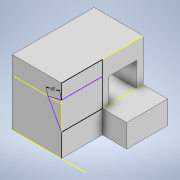
# Autodesk Inventor part: Vỏ
Saved by Autodesk Inventor 2020 (Build 240168000, 168)
## iProperties
Created: 2022-09-23
Part Number: Vỏ
Material: Generic
Document SubType Name: Modeling
Designer: ASUS
Density: 1 g/cm^3
Appearance: Default
Author: ASUS
Autodesk Inventor part; units mm, degrees
ref_plane "YZ Plane" through (0, 0, 0) normal (1, 0, 0) x (0, 1, 0)
ref_plane "XZ Plane" through (0, 0, 0) normal (0, 1, 0) x (-1, 0, 0)
ref_plane "XY Plane" through (0, 0, 0) normal (0, 0, 1) x (1, 0, 0)
sketch "Sketch1" plane through (0, 0, 0) normal (1, 0, 0) x (0, 1, 0)
  line L0 (0, 0) -> (400, 0)
  line L1 (400, 0) -> (400, -500)
  line L2 (400, -500) -> (0, -500)
  line L3 (0, -500) -> (0, 0)
  dimension "d0" = 400
  dimension "d1" = 500
  constraints: 8 end point, 2 parallel, 1 horizontal, 1 perpendicular
  measures "d0" distance of L1.end L2.end
  measures "d1" distance of L0.end L1.end
extrude "Extrusion1" add sketch "Sketch1" against normal blind 300
sketch "Sketch2" plane through (0, 0, 0) normal (1, 0, 0) x (0, 0, -1)
  line L0 (500, 0) -> (0, 0) projected
  line L1 (500, 400) -> (500, 0) projected
  line L2 (250, 0) -> (500, 0)
  line L3 (500, 0) -> (500, 140)
  line L4 (500, 140) -> (250, 140)
  line L5 (250, 140) -> (250, 0)
  dimension "d4" = 140
  constraints: 8 end point, 2 parallel, 1 horizontal, 1 midpoint, 1 perpendicular, 1 point on line
  measures "d4" distance of L3.end L2.end
extrude "Extrusion2" add sketch "Sketch2" along normal blind 150
sketch "Sketch3" plane through (0, 0, 0) normal (1, 0, 0) x (0, 0, -1)
  line L0 (250, 140) -> (250, 0) projected
  line L1 (250, 140) -> (290, 140)
  line L2 (290, 140) -> (290, 290)
  line L3 (290, 290) -> (250, 290)
  line L4 (250, 290) -> (250, 140)
  line L5 (500, 400) -> (500, 0) projected
  line L6 (500, 140) -> (460, 140)
  line L7 (460, 140) -> (460, 290)
  line L8 (460, 290) -> (500, 290)
  line L9 (500, 290) -> (500, 140)
  line L10 (290, 290) -> (460, 290)
  line L11 (290, 140) -> (460, 140)
  line L12 (500, 140) -> (250, 140) projected
  point P0 (0, 0)
  dimension "d7" = 40
  dimension "d8" = 150
  dimension "d9" = 40
  constraints: 20 end point, 4 parallel, 3 horizontal, 3 point on line, 2 perpendicular, 1 collinear
  measures "d7" distance of L3.end L2.end
  measures "d8" distance of L2.end L1.end
  measures "d9" distance of L7.end L8.end
extrude "Extrusion3" cut sketch "Sketch3" against normal blind 290 contours L2 L10 L7 L11
sketch "Sketch4" plane through (0, 0, 0) normal (1, 0, 0) x (0, 0, -1)
  line L0 (0, 400) -> (0, 0) projected
  line L1 (0, 310) -> (250, 310)
  line L2 (250, 310) -> (250, 400)
  line L3 (500, 400) -> (0, 400) projected
  line L4 (0, 400) -> (0, 310)
  line L5 (0, 400) -> (250, 400)
  line L6 (500, 140) -> (250, 140) projected
  line L7 (250, 310) -> (250, 140)
  line L8 (250, 140) -> (0, 140)
  line L9 (0, 0) -> (0, 400) projected
  constraints: 12 end point, 2 perpendicular, 2 point on line, 1 collinear, 1 horizontal, 1 midpoint, 1 parallel
sketch "Sketch5" plane through (0, 0, 0) normal (0, 0, 1) x (1, 0, 0)
  line L0 (0, 400) -> (0, 0) projected
  line L1 (0, 310) -> (-82.6136, 290)
  line L2 (0, 290) -> (-290, 290) projected
  line L3 (0, 0) -> (0, 140) projected
  line L4 (-82.6136, 290) -> (0, 140)
  line L5 (0, 140) -> (0, 0)
  line L6 (150, 0) -> (-300, 0) projected
  dimension "d12" = 85
  constraints: 6 end point, 2 point on line, 1 perpendicular
  measures "d12" distance of L1.start L1.end
body "Solid1"
